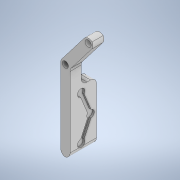
# Autodesk Inventor part: Hank - claw
Saved by Autodesk Inventor 2022 (Build 260153000, 153)
## iProperties
Created: 2022-01-19
Part Number: Hank - claw
Material: Generic
Document SubType Name: Modeling
Designer: chris
Density: 1 g/cm^3
Appearance: Default
Author: chris
Autodesk Inventor part; units mm, degrees
ref_plane "YZ Plane" through (0, 0, 0) normal (1, 0, 0) x (0, 1, 0)
ref_plane "XZ Plane" through (0, 0, 0) normal (0, 1, 0) x (-1, 0, 0)
ref_plane "XY Plane" through (0, 0, 0) normal (0, 0, 1) x (1, 0, 0)
sketch "Sketch1" plane through (0, 0, 0) normal (0, 0, 1) x (1, 0, 0)
  line L0 (0, 0) -> (0, -43.18)
  line L1 (0, 0) -> (12.2773, 16)
  line L2 (0, 0) -> (20.1676, 0) construction
  circle A0 centre (12.2773, 16) radius 1.651
  circle A1 centre (0, 0) radius 1.651
  line L3 (10.0328, 17.2474) -> (-2.54, 0.8622)
  line L4 (-2.54, 0.8622) -> (-2.54, -43.18)
  line L5 (14.063, 14.1549) -> (2.54, -0.8622)
  line L6 (2.54, -0.8622) -> (2.54, -43.18)
  line L7 (10.0328, 17.2474) -> (11.9656, 19.7663)
  line L8 (11.9656, 19.7663) -> (15.9959, 16.6738)
  line L9 (15.9959, 16.6738) -> (14.063, 14.1549)
  line L10 (-2.54, -43.18) -> (2.54, -43.18)
  dimension "d0" = 43.18
  dimension "d1" = 20.1676
  dimension "d2" = 52.5
  dimension "d3" = 3.302
  dimension "d4" = 3.302
  dimension "d5" = 2.54
  dimension "d6" = 2.54
  dimension "d7" = 3.175
  constraints: 22 end point, 2 centre point, 2 coincident, 2 horizontal, 2 perpendicular, 1 equal length, 1 horizontal alignment, 1 vertical, 2 other
  measures "d0" distance of L0.start L0.end
  measures "d1" distance of L0.start L1.end
  measures "d2" angle of L2 L1
  measures "d3" diameter of A0
  measures "d4" diameter of A1
  measures "d5" distance between parallel lines of L1 L3
  measures "d6" distance between parallel lines of L1 L5
  measures "d7" distance of L3.start L7.end
extrude "Extrusion1" add sketch "Sketch1" along normal blind 5.9182
fillet "Fillet1" radius 3.175 6 edges at (11.9656, 19.7663, 2.9591) (15.9959, 16.6738, 2.9591) (-2.54, 0.8622, 2.9591) (2.54, -0.8622, 2.9591) (2.54, -43.18, 2.9591) (-2.54, -43.18, 2.9591)
sketch "Sketch2" plane through (0, 0, 0) normal (0, 0, -1) x (-1, 0, 0)
  line L0 (-2.54, -40.005) -> (-2.54, -1.94) projected
  line L1 (-2.54, -11.43) -> (2.54, -11.43)
  line L2 (2.54, -0.2156) -> (2.54, -40.2701) projected
  arc A0 (-2.54, -40.005) -> (0.635, -43.18) centre (0.635, -40.005) ccw projected
  circle A1 centre (0, 0) radius 1.651 projected
  circle A2 centre (-12.2773, 16) radius 1.651 projected
  arc A3 (0.635, -43.18) -> (2.54, -40.2701) centre (-0.635, -40.2701) ccw projected
  line L3 (2.54, -0.2156) -> (2.54, -40.2701) projected
  arc A4 (2.54, -0.2156) -> (1.8839, 1.7173) centre (-0.635, -0.2156) ccw projected
  line L4 (-10.0328, 17.2474) -> (1.8839, 1.7173) projected
  arc A5 (-10.0328, 17.2474) -> (-14.4845, 17.8335) centre (-12.5517, 15.3146) ccw projected
  arc A6 (-14.4845, 17.8335) -> (-14.2244, 14.3652) centre (-11.7055, 16.298) ccw projected
  line L5 (-3.1961, -0.0072) -> (-14.2244, 14.3652) projected
  arc A7 (-2.54, -1.94) -> (-3.1961, -0.0072) centre (-5.715, -1.94) ccw projected
  line L6 (-2.54, -40.005) -> (-2.54, -1.94) projected
  arc A8 (-2.54, -40.005) -> (0.635, -43.18) centre (0.635, -40.005) ccw projected
  point P0 (0.635, -43.18)
  dimension "d11" = 31.75
  constraints: 2 end point, 2 point on line, 1 horizontal
extrude "Extrusion2" add sketch "Sketch2" along normal blind 8.255 contours L0 L1 L2 A3 A0
fillet "Fillet2" radius 3.175 2 edges at (0, -11.43, 0) (0, -11.43, -8.255)
sketch "Sketch3" plane through (2.54, -40.005, 5.9182) normal (1, 0, 0) x (0, 0, -1)
  circle A0 centre (5.9182, 1.6434) radius 2
  circle A1 centre (5.9182, 25.1399) radius 2
  arc A2 (14.1732, 25.4) -> (10.9982, 28.575) centre (10.9982, 25.4) ccw projected
  line L0 (9.0932, 28.575) -> (10.9982, 28.575) projected
  arc A3 (5.9182, 31.75) -> (9.0932, 28.575) centre (9.0932, 31.75) ccw projected
  line L1 (5.9182, 31.75) -> (5.9182, 38.065) projected
  line L2 (0, 38.065) -> (5.9182, 38.065) projected
  line L3 (0, 0) -> (0, 38.065) projected
  line L4 (0, 0) -> (14.1732, 0) projected
  line L5 (14.1732, 25.4) -> (14.1732, 0) projected
  circle A4 centre (10.9982, 12.7) radius 2
  line L6 (5.9182, 1.6434) -> (10.9982, 12.7)
  line L7 (10.9982, 12.7) -> (5.9182, 25.1399)
  line L8 (4.9924, 24.7618) -> (9.9085, 12.7234)
  line L9 (9.9085, 12.7234) -> (5.0095, 2.0609)
  line L10 (6.844, 25.518) -> (12.0879, 12.6766)
  line L11 (12.0879, 12.6766) -> (6.8269, 1.2259)
  point P0 (5.9182, 40.005)
  point P1 (5.6472, 23.1583)
  point P2 (9.4176, 13.9254)
  point P3 (9.3664, 11.5436)
  point P4 (5.7326, 3.6348)
  point P5 (7.55, 2.7998)
  point P6 (11.1838, 10.7086)
  point P7 (11.2692, 14.6816)
  point P8 (7.4988, 23.9144)
  dimension "d15" = 4
  dimension "d16" = 4
  dimension "d17" = 4
  dimension "d18" = 1
  dimension "d19" = 1
  constraints: 12 end point, 3 centre point, 2 other
  measures "d15" diameter of A0
  measures "d16" diameter of A1
  measures "d17" diameter of A4
  measures "d18" distance between parallel lines of L7 L8
  measures "d19" distance between parallel lines of L7 L10
extrude "Extrusion3" cut sketch "Sketch3" against normal blind 1 contours A0 L4 | A0 L6 A4 L11 | A0 L4 | A0 L9 A4 L6 | L11 L10 A4 | A4 L6 L7 L10 L11 | A4 L9 L8 L7 L6 | A4 L8 L9 | A4 L7 A1 L10 | L8 A1 L7 A4 | A1
body "Solid1"
